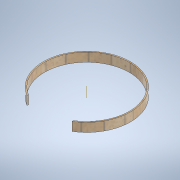
# Autodesk Inventor part: Banding Level A-C Inner
Saved by Autodesk Inventor 2020 (Build 240168000, 168)
## iProperties
Created: 2020-03-10
Part Number: Banding Level A-C Inner
Material: Wood (Maple)
Document SubType Name: Sheet Metal
Designer: Daniel Wikman
Density: 0.67 g/cm^3
Sheet Metal Rule: Default_mm
Appearance: Natural Maple - Glossy Dark Tint
Author: Daniel Wikman
Autodesk Inventor part; units mm, degrees
ref_plane "YZ Plane" through (0, 0, 0) normal (1, 0, 0) x (0, 1, 0)
ref_plane "XZ Plane" through (0, 0, 0) normal (0, 1, 0) x (-1, 0, 0)
ref_plane "XY Plane" through (0, 0, 0) normal (0, 0, 1) x (1, 0, 0)
sketch "Sketch1" plane through (0, 0, 0) normal (0, 1, 0) x (-1, 0, 0)
  circle A0 centre (0, 0) radius 146.07
  circle A1 centre (0, 0) radius 150.07
  dimension "d169" = 292.14
  dimension "d170" = 300.14
  constraints: 2 centre point, 1 coincident
  measures "d169" diameter of A0
  measures "d170" diameter of A1
extrude "Extrusion3" add sketch "Sketch1" along normal blind 30
sketch "Sketch3" plane through (0, 30, 0) normal (0, 1, 0) x (1, 0, 0)
  arc A0 (-116.002, -325.2953) -> (116.0075, -325.2934) centre (0, 0) ccw
  arc A1 (-76.6912, -123.0588) -> (76.6965, -123.0555) centre (0, 0) ccw
  line L0 (-122.1811, -173.696) -> (-161.3589, -227.6196) construction
  line L1 (-116.002, -325.2953) -> (-76.6912, -123.0588)
  line L2 (0, 0) -> (0, -341.2918)
  line L3 (116.0075, -325.2934) -> (76.6965, -123.0555)
  line L4 (161.3912, -227.6651) -> (122.2055, -173.7307) construction
  dimension "d52" = 25
  dimension "d87" = 145
  dimension "d88" = 345.36
  dimension "d89" = 25
  dimension "d90" = 11
  dimension "d91" = 11
  constraints: 8 end point, 4 point on circle, 2 centre point, 1 coincident, 2 other
  measures "d52" angle of L0 L1
  measures "d87" radius of A1
  measures "d88" radius of A0
  measures "d89" angle of L4 L3
  measures "d90" angle of L3 L2
  measures "d91" angle of L1 L2
extrude "Extrusion5" cut sketch "Sketch3" against normal through all
equation "\"BendRadius\" = Thickness"
equation "\"BendReliefWidth\" = Thickness"
equation "\"BendReliefDepth\" = 0.5 * Thickness"
equation "\"CornerReliefSize\" = 4 * Thickness"
equation "\"MinimumRemnant\" = 2 * Thickness"
equation "\"TransitionRadius\" = BendRadius"
equation "\"JacobiRadiusSize\" = BendRadius"
equation "\"GapSize\" = Thickness"
equation "\"Thickness\" = 0.5"
body "Solid3"
